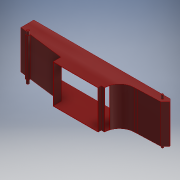
# Autodesk Inventor part: shaker
Saved by Autodesk Inventor 2017 (Build 210142000, 142)
## iProperties
Created: 2017-04-20
Part Number: shaker
Material: Generic
Document SubType Name: Modeling
Designer: master
Density: 1 g/cm^3
Appearance: Reflective - Red
Mass: 1.58424 g
Surface Area: 118.554 cm^2
Volume: 1.58424 cm^3
Author: master
Autodesk Inventor part; units mm, degrees
ref_plane "YZ Plane" through (0, 0, 0) normal (1, 0, 0) x (0, 1, 0)
ref_plane "XZ Plane" through (0, 0, 0) normal (0, 1, 0) x (-1, 0, 0)
sketch "Sketch1" plane through (0, 0, 0) normal (0, 0, 1) x (1, 0, 0)
  line L0 (0, 0) -> (35, 0)
  line L1 (35, 0) -> (35, 2.5)
  line L2 (35, 2.5) -> (37.5, 2.5)
  line L3 (0, 0) -> (0, 6)
  line L4 (-35.5, 20.5) -> (70.5, 20.5)
  line L5 (-35.5, 20.5) -> (-35.5, 10.5)
  line L6 (-35.5, 10.5) -> (0, 6)
  line L7 (70.5, 20.5) -> (72.62132, 18.37868)
  line L8 (70.5, 20.5) -> (73.5, 20.5) construction
  line L9 (72.62132, 18.37868) -> (69.085786, 14.843146)
  line L10 (69.085786, 14.843146) -> (51.399214, 14.234204)
  line L11 (49.236361, 14.133306) -> (49.133306, 14.133306)
  arc A0 (49.133306, 14.133306) -> (37.5, 2.5) centre (49.133306, 2.5) ccw
  line L12 (49.236361, 14.133306) -> (51.399214, 14.234204)
  point P0 (4.506602, 27.156572)
  dimension "d1" = 35
  dimension "d2" = 2.5
  dimension "d3" = 2.5
  dimension "d4" = 6
  dimension "d6" = 106
  dimension "d7" = 20.5
  dimension "d8" = 10
  dimension "d9" = 35.5
  dimension "d10" = 3
  dimension "d11" = 45
  dimension "d12" = 5
  dimension "d18" = 17.68657
  dimension "d19" = 136.972
  dimension "d20" = 11.63331
  dimension "d21" = 2.16285
  constraints: 26 end point, 4 horizontal, 3 perpendicular, 2 point on circle, 2 vertical, 1 centre point, 1 equal length, 1 point on line, 1 tangent
  measures "d1" distance of L0.start L0.end
  measures "d2" distance of L0.end L1.end
  measures "d3" distance of L1.end L2.end
  measures "d4" distance of L0.start L3.end
  measures "d6" distance of L4.start L4.end
  measures "d7" distance from line of L0.start L4
  measures "d8" distance of L4.start L5.end
  measures "d9" distance from line of L0.start L5
  measures "d10" distance of L4.end L7.end
  measures "d11" angle of L7 L8
  measures "d12" distance of L7.end L9.end
  measures "d18" horizontal distance of L9.end L10.end
  measures "d19" angle of L9 L10
  measures "d20" radius of A0
  measures "d21" horizontal distance of L11.start L10.end
extrude "Extrusion1" add sketch "Sketch1" along normal blind 0.24
ref_plane "Work Plane1" through (0, 0, -14.76) normal (0, 0, 1) x (1, 0, 0)
mirror "Mirror1" about plane through (0, 0, -14.76) normal (0, 0, 1) of "Extrusion1"
sketch "Sketch2" plane through (0, 0, 0.24) normal (0, 0, 1) x (1, 0, 0)
  line L0 (51.399214, 14.234204) -> (69.085786, 14.843146)
  line L1 (69.085786, 14.843146) -> (72.62132, 18.37868)
  line L2 (69.085786, 14.843146) -> (72.62132, 18.37868)
  line L3 (72.62132, 18.37868) -> (70.5, 20.5)
  line L4 (72.62132, 18.37868) -> (70.5, 20.5)
  line L5 (70.5, 20.5) -> (70.330294, 20.330294)
  line L6 (70.330294, 20.330294) -> (72.275074, 18.385515)
  line L7 (72.275074, 18.385515) -> (68.87908, 14.989521)
  line L8 (68.87908, 14.989521) -> (68.732704, 14.843146)
  line L9 (68.732704, 14.843146) -> (69.085786, 14.843146)
  point P0 (0, 0)
  dimension "d25" = 0.24
  dimension "d26" = 4.80266
  dimension "d27" = 0.20701
  constraints: 14 end point, 2 collinear, 2 perpendicular, 2 point on line, 1 horizontal, 1 parallel
  measures "d25" distance of L3.end L5.end
  measures "d26" distance of L6.end L7.end
  measures "d27" distance of L7.end L8.end
extrude "Extrusion2" add sketch "Sketch2" against normal blind 30
fillet "Fillet1" radius 0.36 1 edges at (72.6213, 18.3787, -14.76)
sketch "Sketch3" plane through (0, 0, -29.52) normal (0, 0, 1) x (1, 0, 0)
  line L0 (70.5, 20.5) -> (-35.5, 20.5)
  line L1 (-35.5, 20.5) -> (-35.5, 10.5)
  line L2 (-35.5, 13.54528) -> (-35.5, 10.5)
  line L3 (0, 6) -> (0, 0)
  line L4 (-35.5, 10.5) -> (0, 6)
  line L5 (0.24, 0) -> (0.24, 6.211498)
  line L6 (0.24, 6.211498) -> (-35.26, 10.711498)
  line L7 (-35.26, 10.711498) -> (-35.26, 13.54528)
  line L8 (-35.5, 20.5) -> (-35.5, 10.5)
  line L9 (-35.5, 20.5) -> (-35.26, 20.5)
  line L10 (70.5, 20.5) -> (-35.5, 20.5)
  line L11 (0, 6) -> (0, 0)
  line L12 (0, 0) -> (0.24, 0)
  line L13 (0, 0) -> (35, 0)
  line L14 (-35.5, 13.54528) -> (-35.5, 13.866774)
  line L15 (-34.424598, 13.866774) -> (-35.5, 13.866774)
  line L16 (-34.424598, 13.866774) -> (-33.817651, 10.528665)
  line L17 (-35.26, 13.54528) -> (-34.628374, 13.54528)
  line L18 (-34.628374, 13.54528) -> (-34.086068, 10.56269)
  dimension "d31" = 0.24
  constraints: 24 end point, 4 point on line, 2 collinear, 1 horizontal, 1 parallel, 1 perpendicular, 1 vertical, 1 other
  measures "d31" distance between parallel lines of L4 L6
extrude "Extrusion3" add sketch "Sketch3" along normal up to next
fillet "Fillet2" radius 0.36 1 edges at (-34.4246, 13.8668, -14.76)
fillet "Fillet3" radius 0.2 1 edges at (-35.5, 13.8668, -14.76)
fillet "Fillet4" radius 0.4 2 edges at (-35.5, 20.5, -29.64) (-35.5, 20.5, 0.12)
sketch "Sketch4" plane through (0, 0, 0.24) normal (0, 0, 1) x (1, 0, 0)
  line L0 (35, 0) -> (35, 2.5) projected
  line L1 (35, 2.5) -> (37.5, 2.5) projected
  line L2 (34.76, 0) -> (34.76, 2.74)
  line L3 (34.76, 2.74) -> (37.5, 2.74)
  line L4 (37.5, 2.5) -> (37.5, 2.74)
  line L5 (35, 0) -> (34.76, 0)
  point P0 (0, 0)
  dimension "d37" = 0.24
  constraints: 8 end point, 1 perpendicular, 1 vertical, 1 other
  measures "d37" distance between parallel lines of L0 L2
extrude "Extrusion4" add sketch "Sketch4" against normal up to next
fillet "Fillet5" radius 0.24 1 edges at (34.76, 2.74, -14.76)
sketch "Sketch6" plane through (0, 0, 0.24) normal (0, 0, 1) x (1, 0, 0)
  line L0 (51.399214, 14.234204) -> (69.085786, 14.843146)
  line L1 (49.236361, 14.133306) -> (51.399214, 14.234204)
  arc A0 (49.133306, 14.133306) -> (37.5, 2.5) centre (49.133306, 2.5) ccw
  line L2 (49.133306, 14.133306) -> (49.236361, 14.133306)
  line L3 (69.334491, 15.091851) -> (51.389493, 14.474011)
  line L4 (51.389493, 14.474011) -> (49.230766, 14.373306)
  line L5 (49.230766, 14.373306) -> (49.133306, 14.373306)
  arc A1 (49.133306, 14.373306) -> (37.821602, 6.108428) centre (49.133306, 2.5) ccw
  line L6 (69.085786, 14.843146) -> (72.366762, 18.124121)
  line L7 (37.821602, 6.108428) -> (38.073783, 6.108428)
  point P0 (0, 0)
  dimension "d48" = 0.24
  dimension "d49" = 0.24
  dimension "d50" = 0.24
  dimension "d51" = 0.25218
  constraints: 8 end point, 3 point on circle, 1 centre point, 1 horizontal, 1 point on line, 1 other
  measures "d48" distance between parallel lines of L1 L4
  measures "d49" distance between parallel lines of L3 L0
  measures "d50" radial gap between concentric circles of A0 A1
  measures "d51" distance of L7.start L7.end
extrude "Extrusion6" add sketch "Sketch6" against normal up to next
sketch "Sketch7" plane through (0, 0, 0.24) normal (0, 0, 1) x (1, 0, 0)
  arc A0 (72.366762, 18.124121) -> (72.366762, 18.633238) centre (72.112203, 18.37868) ccw
  circle A1 centre (67.472203, 17.647407) radius 0.75
  point P0 (0, 0)
  dimension "d56" = 1.5
  constraints: 1 centre point
  measures "d56" diameter of A1
extrude "Extrusion7" add sketch "Sketch7" along normal blind 3 and the other way blind 33
chamfer "Chamfer1" distance 0.23 angle 45 2 edges at (66.7222, 17.6474, -32.76) (66.7222, 17.6474, 3.24)
sketch "Sketch8" plane through (35, 0, -29.76) normal (0, 0, -1) x (-1, 0, 0)
  line L0 (70.5, 10.5) -> (35, 6)
  line L1 (62.016409, 9.424615) -> (62.016409, 7.424615)
  line L2 (62.016409, 7.424615) -> (64.016409, 7.424615)
  line L3 (64.016409, 7.424615) -> (64.016409, 9.678136)
  line L4 (62.016409, 9.424615) -> (64.016409, 9.678136)
  point P0 (35, 0)
  dimension "d64" = 2
  dimension "d65" = 2
  constraints: 8 end point, 2 perpendicular, 2 point on line, 1 vertical
  measures "d64" distance of L1.start L1.end
  measures "d65" distance of L1.end L2.end
extrude "Extrusion8" add sketch "Sketch8" against normal blind 30
sketch "Sketch9" plane through (0, 0, 0.24) normal (0, 0, 1) x (1, 0, 0)
  line L0 (-29.016409, 9.678136) -> (-29.016409, 7.424615)
  line L1 (-29.016409, 7.424615) -> (-27.016409, 7.424615)
  line L2 (-27.016409, 7.424615) -> (-27.016409, 9.424615)
  circle A0 centre (-28.016409, 8.424615) radius 1
  point P0 (0, 0)
  constraints: 3 tangent, 1 centre point
extrude "Extrusion9" add sketch "Sketch9" along normal blind 3 and the other way blind 33 contours A0
chamfer "Chamfer2" distance 0.23 angle 45 2 edges at (-29.0164, 8.4246, 3.24) (-29.0164, 8.4246, -32.76)
body "Solid1"
